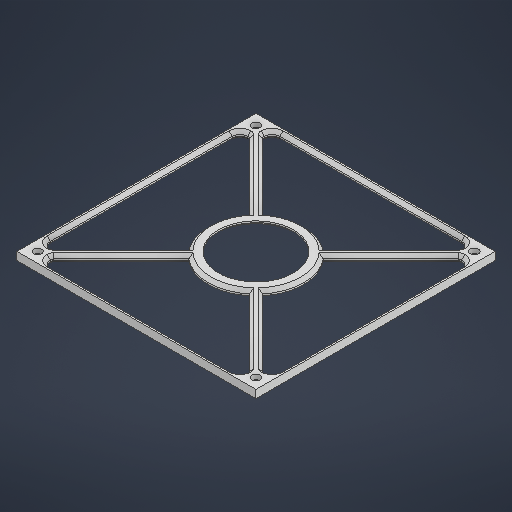
# Autodesk Inventor part: upLid
Saved by Autodesk Inventor 2025.1 (Build 291241000, 241)
## iProperties
Created: 2025-11-23
Part Number: upLid
Material: Типовые
Document SubType Name: Modeling
Designer: bogda
Density: 1 g/cm^3
Appearance: По умолчанию
Author: bogda
Autodesk Inventor part; units mm, degrees
ref_plane "YZ Plane" through (0, 0, 0) normal (1, 0, 0) x (0, 1, 0)
ref_plane "XZ Plane" through (0, 0, 0) normal (0, 1, 0) x (-1, 0, 0)
ref_plane "XY Plane" through (0, 0, 0) normal (0, 0, 1) x (1, 0, 0)
sketch "Эскиз1" plane through (0, 0, 0) normal (0, 1, 0) x (-1, 0, 0)
  line L0 (0, 0) -> (150, 0)
  line L1 (150, 0) -> (150, -150)
  line L2 (150, -150) -> (0, -150)
  line L3 (0, -150) -> (0, 0)
  line L4 (150, 0) -> (137, 0)
  line L5 (137, -8) -> (137, -8)
  line L6 (142, -13) -> (142, -13)
  line L7 (150, -13) -> (150, 0)
  line L8 (150, -150) -> (137, -150)
  line L9 (137, -142) -> (137, -142)
  line L10 (142, -137) -> (142, -137)
  line L11 (150, -137) -> (150, -150)
  line L12 (0, 0) -> (13, 0)
  line L13 (13, -8) -> (13, -8)
  line L14 (8, -13) -> (8, -13)
  line L15 (0, -13) -> (0, 0)
  line L16 (0, -150) -> (13, -150)
  line L17 (13, -142) -> (13, -142)
  line L18 (8, -137) -> (8, -137)
  line L19 (0, -137) -> (0, -150)
  circle A0 centre (143.5, -6.5) radius 2.6
  circle A1 centre (143.5, -143.5) radius 2.6
  circle A2 centre (6.5, -143.5) radius 2.6
  circle A3 centre (6.5, -6.5) radius 2.6
  line L20 (18, -3) -> (132, -3)
  line L21 (147, -18) -> (147, -132)
  line L22 (132, -147) -> (18, -147)
  line L23 (3, -132) -> (3, -18)
  arc A4 (18, -3) -> (13.0014, -7.8829) centre (18, -8) ccw
  arc A5 (7.8829, -13.0014) -> (3, -18) centre (8, -18) ccw
  arc A6 (3, -132) -> (7.8829, -136.9986) centre (8, -132) ccw
  arc A7 (13.0014, -142.1171) -> (18, -147) centre (18, -142) ccw
  arc A8 (132, -147) -> (136.9986, -142.1171) centre (132, -142) ccw
  arc A9 (142.1171, -136.9986) -> (147, -132) centre (142, -132) ccw
  arc A10 (147, -18) -> (142.1171, -13.0014) centre (142, -18) ccw
  arc A11 (136.9986, -7.8829) -> (132, -3) centre (132, -8) ccw
  circle A12 centre (75, -75) radius 30
  line L24 (136.4134, -140.656) -> (93.9856, -98.2282)
  line L25 (140.656, -136.4134) -> (98.2282, -93.9856)
  line L26 (51.7718, -56.0144) -> (9.344, -13.5866)
  line L27 (56.0144, -51.7718) -> (13.5866, -9.344)
  line L28 (136.4134, -9.344) -> (93.9856, -51.7718)
  line L29 (140.656, -13.5866) -> (98.2282, -56.0144)
  line L30 (56.0144, -98.2282) -> (13.5866, -140.656)
  line L31 (51.7718, -93.9856) -> (9.344, -136.4134)
  arc A13 (136.9986, -142.1171) -> (136.4134, -140.656) centre (134.9992, -142.0702) ccw
  arc A14 (140.656, -136.4134) -> (142.1171, -136.9986) centre (142.0702, -134.9992) ccw
  arc A15 (13.5866, -140.656) -> (13.0014, -142.1171) centre (15.0008, -142.0702) ccw
  arc A16 (7.8829, -136.9986) -> (9.344, -136.4134) centre (7.9298, -134.9992) ccw
  arc A17 (9.344, -13.5866) -> (7.8829, -13.0014) centre (7.9298, -15.0008) ccw
  arc A18 (13.0014, -7.8829) -> (13.5866, -9.344) centre (15.0008, -7.9298) ccw
  arc A19 (136.4134, -9.344) -> (136.9986, -7.8829) centre (134.9992, -7.9298) ccw
  arc A20 (142.1171, -13.0014) -> (140.656, -13.5866) centre (142.0702, -15.0008) ccw
  circle A21 centre (75, -75) radius 23.5
  dimension "d19" = 60
  dimension "d0" = 150
  dimension "d1" = 150
  dimension "d11" = 5.2
  dimension "d12" = 5.2
  dimension "d14" = 3
  dimension "d15" = 3
  dimension "d16" = 3
  dimension "d17" = 3
  dimension "d18" = 5
  dimension "d25" = 2
  dimension "d26" = 2
  dimension "d27" = 2
  constraints: 64 end point, 40 point on circle, 32 tangent, 21 centre point, 14 parallel, 12 equal radius, 8 point on line, 5 horizontal, 5 perpendicular, 1 coincident, 10 other
  measures "d0" distance of L1.end L2.end
  measures "d1" distance of L0.end L1.end
  measures "d11" diameter of A1
  measures "d12" diameter of A2
  measures "d14" distance between parallel lines of L0 L20
  measures "d15" distance between parallel lines of L1 L21
  measures "d16" distance between parallel lines of L2 L22
  measures "d17" distance between parallel lines of L3 L23
  measures "d18" radius of A4
  measures "d25" radius of A13
  measures "d26" radius of A15
  measures "d27" radius of A17
extrude "Выдавливание1" add sketch "Эскиз1" along normal blind 3 contours L0 L1 L2 L3 | A12
extrude "Выдавливание2" add sketch "Эскиз1" against normal blind 2 contours L0 L1 L2 L3 | A0 | A1 | A2 | A3
chamfer "Фаска1" distance 2 angle 45 4 edges at (-53.7868, 0, -53.7868) (-53.7868, 0, -96.2132) (-96.2132, 0, -53.7868) (-96.2132, 0, -96.2132)
chamfer "Фаска2" distance 2 angle 45 4 edges at (-105, 3, -75) (-75, 3, -45) (-45, 3, -75) (-75, 3, -105)
chamfer "Фаска3" distance 2 angle 45 28 edges at (-35.5115, 3, -31.2688) (-13.1442, 3, -8.6734) (-14.5061, 3, -4.4233) (-75, 3, -3) (-135.4939, 3, -4.4233) (-136.8558, 3, -8.6734) (-114.4885, 3, -31.2688) (-31.2688, 3, -35.5115) (-8.6734, 3, -13.1442) (-4.4233, 3, -14.5061) (-3, 3, -75) (-4.4233, 3, -135.4939) (-8.6734, 3, -136.8558) (-31.2688, 3, -114.4885) (-75, 3, -147) (-14.5061, 3, -145.5767) (-13.1442, 3, -141.3266) (-35.5115, 3, -118.7312) (-135.4939, 3, -145.5767) (-136.8558, 3, -141.3266) (-114.4885, 3, -118.7312) (-118.7312, 3, -35.5115) (-141.3266, 3, -13.1442) (-145.5767, 3, -14.5061) (-147, 3, -75) (-145.5767, 3, -135.4939) (-141.3266, 3, -136.8558) (-118.7312, 3, -114.4885)
chamfer "Фаска4" distance 2 angle 45 29 edges at (-119.4421, -2, -34.8005) (-141.3266, -2, -13.1442) (-145.5767, -2, -14.5061) (-147, -2, -75) (-145.5767, -2, -135.4939) (-141.3266, -2, -136.8558) (-119.4421, -2, -115.1995) (-115.1995, -2, -119.4421) (-136.8558, -2, -141.3266) (-135.4939, -2, -145.5767) (-75, -2, -147) (-14.5061, -2, -145.5767) (-13.1442, -2, -141.3266) (-34.8005, -2, -119.4421) (-30.5579, -2, -34.8005) (-8.6734, -2, -13.1442) (-4.4233, -2, -14.5061) (-3, -2, -75) (-4.4233, -2, -135.4939) (-8.6734, -2, -136.8558) (-30.5579, -2, -115.1995) (-34.8005, -2, -30.5579) (-13.1442, -2, -8.6734) (-14.5061, -2, -4.4233) (-75, -2, -3) (-135.4939, -2, -4.4233) (-136.8558, -2, -8.6734) (-115.1995, -2, -30.5579) (-51.5, 0, -75)
